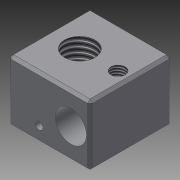
# Autodesk Inventor part: E3D_Heaterblock
Saved by Autodesk Inventor 2014 (Build 180170000, 170)
## iProperties
Created: 2014-09-30
Part Number: E3D_Heaterblock
Material: Generic
Document SubType Name: Modeling
Designer: ThatOtherGuy
Density: 1 g/cm^3
Appearance: Default
Author: ThatOtherGuy
Autodesk Inventor part; units mm, degrees
ref_plane "YZ Plane" through (0, 0, 0) normal (1, 0, 0) x (0, 1, 0)
ref_plane "XZ Plane" through (0, 0, 0) normal (0, 1, 0) x (-1, 0, 0)
ref_plane "XY Plane" through (0, 0, 0) normal (0, 0, 1) x (1, 0, 0)
sketch "Sketch1" plane through (0, 0, 0) normal (0, 0, 1) x (1, 0, 0)
  line L0 (0, 0) -> (16, 0)
  line L1 (16, 0) -> (16, 16)
  line L2 (16, 16) -> (0, 16)
  line L3 (0, 16) -> (0, 0)
  dimension "d0" = 16
  dimension "d1" = 16
  constraints: 8 end point, 2 parallel, 1 horizontal, 1 perpendicular
  measures "d0" distance of L1.end L2.end
  measures "d1" distance of L2.end L0.start
extrude "Extrusion1" add sketch "Sketch1" along normal blind 12
sketch "Sketch3" plane through (0, 0, 0) normal (0, -1, 0) x (1, 0, 0)
  line L0 (0, 0) -> (16, 0) projected
  line L1 (0, 0) -> (0, 12) projected
  circle A0 centre (6, 3) radius 0.75
  circle A1 centre (12.25, 6) radius 3.05
  dimension "d10" = 6.1
  dimension "d11" = 1.5
  dimension "d12" = 3
  dimension "d13" = 6
  dimension "d14" = 6
  dimension "d15" = 12.25
  constraints: 2 centre point
  measures "d10" diameter of A1
  measures "d11" diameter of A0
  measures "d12" distance from line of L0 A0.centre
  measures "d13" distance from line of L1 A0.centre
  measures "d14" distance from line of A1.centre L0
  measures "d15" distance from line of L1 A1.centre
sketch "Sketch2" plane through (0, 0, 12) normal (0, 0, 1) x (1, 0, 0)
  line L0 (0, 16) -> (0, 0) projected
  circle A0 centre (6, 8) radius 3
  circle A1 centre (13.5, 8) radius 1.4
  point P0 (0, 8)
  dimension "d4" = 13.5
  dimension "d5" = 6
  dimension "d6" = 6
  dimension "d7" = 2.8
  constraints: 2 centre point, 2 horizontal alignment, 1 midpoint
  measures "d4" distance from line of L0 A1.centre
  measures "d5" distance from line of L0 A0.centre
  measures "d6" diameter of A0
  measures "d7" diameter of A1
chamfer "Chamfer1" distance 0.5 angle 45 12 edges at (0, 0, 6) (8, 0, 12) (0, 8, 12) (8, 16, 12) (0, 16, 6) (0, 8, 0) (8, 16, 0) (8, 0, 0) (16, 8, 0) (16, 8, 12) (16, 0, 6) (16, 16, 6)
extrude "Extrusion4" cut sketch "Sketch3" against normal up to next
extrude "Extrusion5" cut sketch "Sketch2" against normal up to next
thread "Thread1" size "M6x1" class "6H" standard "ANSI Metric M Profile" full length
thread "Thread2" size "M3x0.5" class "6H" standard "ANSI Metric M Profile" full length
body "Solid1"
